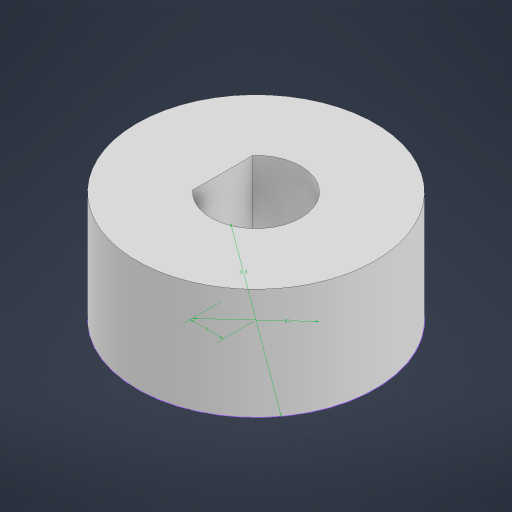
# Autodesk Inventor part: Motor_Couple
Saved by Autodesk Inventor 2023 (Build 270158000, 158)
## iProperties
Created: 2023-11-17
Part Number: Motor_Couple
Material: Generic
Document SubType Name: Modeling
Designer: Abhinav
Density: 1 g/cm^3
Appearance: Default
Author: Abhinav
Autodesk Inventor part; units mm, degrees
ref_plane "YZ Plane" through (0, 0, 0) normal (1, 0, 0) x (0, 1, 0)
ref_plane "XZ Plane" through (0, 0, 0) normal (0, 1, 0) x (-1, 0, 0)
ref_plane "XY Plane" through (0, 0, 0) normal (0, 0, 1) x (1, 0, 0)
sketch "Sketch1" plane through (0, 0, 0) normal (0, 1, 0) x (-1, 0, 0)
  arc A0 (3, 2.7208) -> (3, -2.7208) centre (0, 0) ccw
  line L0 (0, 0) -> (3, 0)
  line L1 (3, 0) -> (3, -2.7208)
  line L2 (3, 0) -> (3, 2.7208)
  circle A1 centre (0, 0) radius 10.75
  dimension "d1" = 8.1
  dimension "d2" = 3
  dimension "d11" = 21.5
  constraints: 6 end point, 2 centre point, 2 point on circle, 1 coincident, 1 horizontal, 1 perpendicular, 1 vertical
  measures "d1" diameter of A0
  measures "d2" distance of L0.start L0.end
  measures "d11" diameter of A1
extrude "Extrusion1" add sketch "Sketch1" along normal blind 10
body "Solid1"
